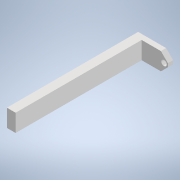
# Autodesk Inventor part: rotator_squarer
Saved by Autodesk Inventor 2022 (Build 260153000, 153)
## iProperties
Created: 2021-07-13
Part Number: rotator_squarer
Material: Generic
Document SubType Name: Modeling
Designer: dsdan
Density: 1 g/cm^3
Appearance: Default
Author: dsdan
Autodesk Inventor part; units mm, degrees
ref_plane "YZ Plane" through (0, 0, 0) normal (1, 0, 0) x (0, 1, 0)
ref_plane "XZ Plane" through (0, 0, 0) normal (0, 1, 0) x (-1, 0, 0)
ref_plane "XY Plane" through (0, 0, 0) normal (0, 0, 1) x (1, 0, 0)
sketch "Sketch1" plane through (0, 0, 0) normal (0, 1, 0) x (-1, 0, 0)
  line L0 (0, 0) -> (10, 0)
  line L1 (10, 0) -> (10, 150)
  line L2 (10, 150) -> (0, 150)
  line L3 (0, 150) -> (0, 0)
  line L4 (0, 6) -> (-30, 6)
  line L5 (-30, 6) -> (-30, 0)
  line L6 (-30, 0) -> (0, 0)
  line L7 (0, 0) -> (0, 6)
  dimension "d0" = 10
  dimension "d1" = 150
  dimension "d2" = 30
  dimension "d3" = 6
  constraints: 16 end point, 4 parallel, 2 horizontal, 2 perpendicular, 2 point on line
  measures "d0" distance between parallel lines of L3 L1
  measures "d1" distance between parallel lines of L2 L0
  measures "d2" distance of L4.start L4.end
  measures "d3" distance between parallel lines of L6 L4
extrude "Extrusion1" add sketch "Sketch1" along normal blind 20
sketch "Sketch2" plane through (0, 0, 6) normal (0, 0, 1) x (1, 0, 0)
  circle A0 centre (25.543, 10) radius 3.1
  line L0 (30, 0) -> (30, 20) projected
  point P0 (0, 0)
  point P1 (30, 10)
  dimension "d6" = 6.2
  dimension "d9" = 4.457
  constraints: 1 centre point, 1 horizontal alignment, 1 midpoint
  measures "d6" diameter of A0
  measures "d9" distance from line of L0 A0.centre
extrude "Extrusion2" cut sketch "Sketch2" against normal through all
chamfer "Chamfer1" distance 8 angle 45 2 edges at (30, 0, 3) (30, 20, 3)
body "Solid1"
